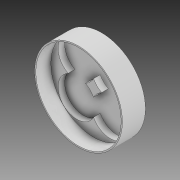
# Autodesk Inventor part: Base
Saved by Autodesk Inventor 2020 (Build 240168000, 168)
## iProperties
Created: 2021-04-03
Part Number: Base
Material: Generic
Document SubType Name: Modeling
Designer: DDeGo
Density: 1 g/cm^3
Appearance: Default
Author: DDeGo
Autodesk Inventor part; units mm, degrees
ref_plane "YZ Plane" through (0, 0, 0) normal (1, 0, 0) x (0, 1, 0)
ref_plane "XZ Plane" through (0, 0, 0) normal (0, 1, 0) x (-1, 0, 0)
ref_plane "XY Plane" through (0, 0, 0) normal (0, 0, 1) x (1, 0, 0)
sketch "Sketch1" plane through (0, 0, 0) normal (0, 0, 1) x (1, 0, 0)
  circle A0 centre (0, 0) radius 50 construction
  circle A1 centre (0, 0) radius 52.5
  dimension "d0" = 100
  dimension "d1" = 105
  constraints: 2 centre point, 2 coincident
  measures "d0" diameter of A0
  measures "d1" diameter of A1
extrude "Extrusion1" add sketch "Sketch1" along normal blind 1.5
sketch "Sketch2" plane through (0, 0, 1.5) normal (0, 0, 1) x (1, 0, 0)
  line L0 (-20, -20) -> (20, -20) construction
  line L1 (20, -20) -> (20, 20) construction
  line L2 (20, 20) -> (-20, 20) construction
  line L3 (-20, 20) -> (-20, -20) construction
  line L4 (-20, -20) -> (20, 20) construction
  line L5 (20, -20) -> (-20, 20) construction
  circle A0 centre (-20, 20) radius 22.5
  circle A1 centre (20, 20) radius 22.5
  circle A2 centre (20, -20) radius 22.5
  circle A3 centre (-20, -20) radius 22.5
  circle A4 centre (0, 0) radius 52.5 projected
  point P0 (-9.6922, 0)
  point P1 (0, -9.6922)
  point P2 (9.6922, 0)
  point P3 (0, 9.6922)
  point P4 (0, -30.3078)
  point P5 (-30.3078, 0)
  point P6 (0, 30.3078)
  point P7 (30.3078, 0)
  dimension "d4" = 45
  dimension "d5" = 40
  constraints: 12 end point, 4 centre point, 4 coincident, 3 equal radius, 2 midpoint, 2 parallel, 2 perpendicular, 1 horizontal
  measures "d4" diameter of A1
  measures "d5" distance of L0.end L1.end
extrude "Extrusion2" add sketch "Sketch2" along normal blind 8 contours A1 A2 A3 A0 | A4
sketch "Sketch3" plane through (0, 0, 9.5) normal (0, 0, 1) x (1, 0, 0)
  circle A0 centre (0, 0) radius 51
  circle A1 centre (0, 0) radius 52.5 projected
  dimension "d8" = 1.5
  constraints: 1 centre point, 1 coincident
  measures "d8" radial gap between concentric circles of A1 A0
extrude "Extrusion3" add sketch "Sketch3" along normal blind 18
sketch "Sketch4" plane through (0, 0, 0) normal (0, 0, -1) x (-1, 0, 0)
  line L0 (0, 0) -> (42, 0) construction
  circle A0 centre (42, 0) radius 6
  circle A1 centre (0, 42) radius 6
  circle A2 centre (-42, 0) radius 6
  circle A3 centre (0, -42) radius 6
  dimension "d11" = 12
  dimension "d12" = 42
  dimension "d15" = 360
  constraints: 4 centre point, 2 end point, 1 coincident, 1 horizontal, 9 other
  measures "d11" diameter of A0
  measures "d12" distance of L0.start L0.end
extrude "Extrusion4" cut sketch "Sketch4" against normal blind 2
body "Solid1"
